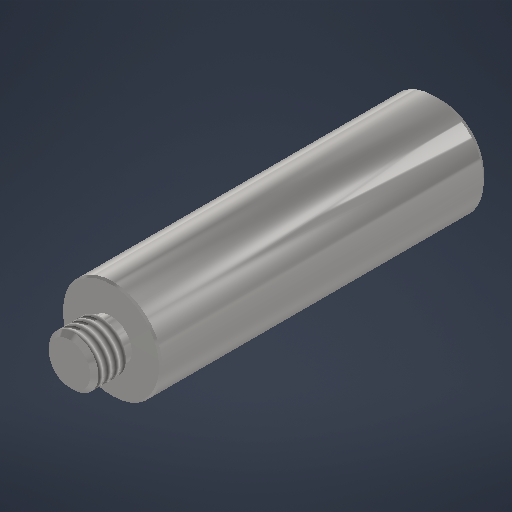
# Autodesk Inventor part: rod
Saved by Autodesk Inventor 2026 (Build 300175050, 175E)
## iProperties
Created: 2025-07-09
Part Number: rod
Material: ステンレス鋼
Document SubType Name: Modeling
Designer: jin20
Density: 8 g/cm^3
Appearance: 半つや出し
Author: jin20
Autodesk Inventor part; units mm, degrees
ref_plane "YZ Plane" through (0, 0, 0) normal (1, 0, 0) x (0, 1, 0)
ref_plane "XZ Plane" through (0, 0, 0) normal (0, 1, 0) x (-1, 0, 0)
ref_plane "XY Plane" through (0, 0, 0) normal (0, 0, 1) x (1, 0, 0)
sketch "スケッチ1" plane through (0, 0, 0) normal (0, 1, 0) x (-1, 0, 0)
  circle A0 centre (28.5834, 76.5526) radius 3
  circle A1 centre (28.5834, 76.5526) radius 6
  line L0 (22.5834, 53.97) -> (22.5834, 15.17)
  line L1 (34.5834, 15.17) -> (34.5834, 53.97)
  line L2 (34.3834, 54.17) -> (22.7834, 54.17)
  line L3 (34.5834, 53.97) -> (22.5834, 53.97)
  line L4 (31.0834, 59.17) -> (31.5834, 58.67)
  line L5 (31.5834, 58.67) -> (31.5834, 55.37)
  line L6 (31.0834, 55.37) -> (31.0834, 54.17)
  line L7 (25.5834, 55.37) -> (25.5834, 58.67)
  line L8 (25.5834, 58.67) -> (26.0834, 59.17)
  line L9 (22.7834, 54.17) -> (22.5834, 53.97)
  line L10 (26.0834, 54.17) -> (26.0834, 55.37)
  line L11 (26.0834, 59.17) -> (31.0834, 59.17)
  line L12 (31.5834, 55.37) -> (25.5834, 55.37)
  line L13 (25.5834, 58.67) -> (31.5834, 58.67)
  circle A2 centre (28.5834, 49.17) radius 2
  line L14 (34.5834, 53.97) -> (34.3834, 54.17)
  line L15 (23.5834, 14.17) -> (33.5834, 14.17)
  line L16 (34.5834, 15.17) -> (22.5834, 15.17)
  line L17 (22.5834, 15.17) -> (23.5834, 14.17)
  line L18 (33.5834, 14.17) -> (34.5834, 15.17)
  line L19 (22.2839, 93.8265) -> (34.3573, 93.8265)
  circle A3 centre (28.5834, 76.5526) radius 2.5
  line L20 (31.0834, 59.17) -> (31.0834, 55.37)
  line L21 (26.0834, 55.37) -> (26.0834, 59.17)
  line L22 (28.5834, 59.8312) -> (28.5834, 13.6756)
  line L23 (28.5834, 83.2838) -> (28.5834, 69.8215)
  line L24 (35.6367, 76.5526) -> (21.5301, 76.5526)
  line L25 (31.4196, 49.17) -> (25.9045, 49.17)
  point P0 (0, 0)
  point P1 (46.1521, 14.1073)
  point P2 (22.8046, 94.5122)
  point P3 (28.5834, 14.17)
  point P4 (28.5834, 59.17)
  constraints: 52 end point, 4 centre point, 2 other
revolve "回転1" add sketch "スケッチ1" angle 360 about axis through (-28.5834, 0, 59.8312) along (0, 0, -1) picked at (29.9, 49.3183) picked at (29.9, 49.0217) contours L22 L2 L14 L3 | L3 L1 L16 L22 A2 | L16 L18 L15 L22 | L22 L12 L6 L2 | A2 L25 L22 | L22 L25 A2 | L22 L13 L20 L12 | L20 L13 L5 L12 | L22 L11 L20 L13 | L20 L4 L13
thread "ねじ1" size "M6x1" class "6g" standard "ANSI Metric M Profile" full length
